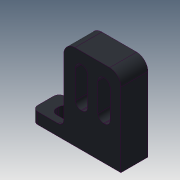
# Autodesk Inventor part: J005556
Saved by Autodesk Inventor 2015 SP1 (Build 190203100, 203)
## iProperties
Created: 2015-12-16
Material: VERO BLACK
Vendor: HHMI: JRC - ID&F
Document SubType Name: Modeling
Designer: ARNOLDJ
Density: 1.17 g/cm^3
Appearance: Black Anodize
Description: NRB ADAPTER ML BRACKET
Project: COMMON
Part Number: J005556
RuleStatus: InUse
AfterDocSave0: file://Part Number Cleaner
LAB/DEPT: COMMON
REQUESTING SCIENTIST: COMMON
SURFACE ROUGHNESS: N/A
DESIGN DEPARTMENT: HHMI: JRC - ID&F
SPECIAL FINISH: NONE
ALTERED ITEM PART NUMBER: N/A
ALTERED ITEM VENDOR: N/A
ALTERED ITEM DESCRIPTION: N/A
Revision Number: -
Autodesk Inventor part; units mm, degrees
sketch "Sketch1" plane through (0, 0, 0) normal (0, 0, 1) x (1, 0, 0)
  line L0 (0, 57.912) -> (0, -9.652) projected
  line L1 (-63.881, 0) -> (36.576, 0) projected
  line L2 (22.225, 48.26) -> (-27.94, 48.26)
  line L3 (-27.94, 48.26) -> (-27.94, 0)
  line L4 (-27.94, 0) -> (22.225, 0)
  line L5 (22.225, 0) -> (22.225, 48.26)
  line L6 (0, 48.26) -> (0, 0) construction
  line L7 (12.7, 48.26) -> (12.7, 0) construction
  line L8 (3.429, 19.305) -> (-3.429, 19.305)
  line L9 (-3.429, 19.305) -> (-3.429, 41.655)
  line L10 (-3.429, 41.655) -> (3.429, 41.655)
  line L11 (3.429, 41.655) -> (3.429, 19.305)
  line L12 (3.429, 19.305) -> (-3.429, 41.655) construction
  line L13 (-3.429, 19.305) -> (3.429, 41.655) construction
  line L14 (16.129, 19.305) -> (9.271, 19.305)
  line L15 (9.271, 19.305) -> (9.271, 41.655)
  line L16 (9.271, 41.655) -> (16.129, 41.655)
  line L17 (16.129, 41.655) -> (16.129, 19.305)
  line L18 (16.129, 19.305) -> (9.271, 41.655) construction
  line L19 (9.271, 19.305) -> (16.129, 41.655) construction
  circle A0 centre (0, 38.48) radius 3.175 construction
  circle A1 centre (0, 30.48) radius 3.175 construction
  line L20 (-27.94, 0) -> (-49.53, 0)
  line L21 (-49.53, 0) -> (-49.53, 7.62)
  line L22 (-49.53, 7.62) -> (-27.94, 7.62)
  line L23 (-27.94, 7.62) -> (-27.94, 0)
  line L24 (-3.9178, 6.35) -> (-23.2802, 6.35)
  line L25 (-23.2802, 6.35) -> (-23.2802, 13.335)
  line L26 (-23.2802, 13.335) -> (-3.9178, 13.335)
  line L27 (-3.9178, 13.335) -> (-3.9178, 6.35)
  line L28 (-3.9178, 6.35) -> (-23.2802, 13.335) construction
  line L29 (-23.2802, 6.35) -> (-3.9178, 13.335) construction
  line L30 (-23.2802, 13.335) -> (-17.0915, 20.955)
  line L31 (-17.0915, 20.955) -> (-10.1065, 20.955)
  line L32 (-10.1065, 20.955) -> (-3.9178, 13.335)
  line L33 (-13.599, 9.8425) -> (-13.599, 20.955) construction
  circle A2 centre (0, 22.48) radius 6.35 construction
  point P0 (0, 0)
  point P1 (0, 25.4)
  point P2 (0, 30.48)
  point P3 (12.7, 30.48)
  point P4 (12.7, 30.48)
  dimension "d0" = 48.26
  dimension "d2" = 6.858
  dimension "d3" = 0
  dimension "d5" = 6.35
  dimension "d6" = 8
  dimension "d27" = 12.7
  dimension "d56" = 41.655
  dimension "d57" = 6.605
  dimension "d58" = 30.48
  dimension "d59" = 7.62
  dimension "d60" = 21.59
  dimension "d61" = 6.985
  dimension "d62" = 6.35
  dimension "d64" = 13.599
  dimension "d81" = 22.225
  dimension "d82" = 27.94
  dimension "d84" = 6.985
  dimension "d85" = 3.4925
  dimension "d86" = 7.62
  dimension "d104" = 12.7
  dimension "d105" = 8
  dimension "d119" = 13.599
  constraints: 64 end point, 10 parallel, 10 point on line, 9 midpoint, 8 perpendicular, 6 horizontal, 3 centre point, 2 coincident, 2 equal length, 1 equal radius, 1 horizontal alignment, 1 tangent
  measures "d0" distance of L2.end L3.end
  measures "d2" distance of L9.end L10.end
  measures "d3" distance between parallel lines of L0 L6
  measures "d5" diameter of A0
  measures "d6" distance of A0.centre A1.centre
  measures "d27" distance of point (0, 30.48) point (12.7, 30.48)
  measures "d56" distance between parallel lines of L4 L10
  measures "d57" distance between parallel lines of L10 L2
  measures "d58" distance from line of L1 A1.centre
  measures "d59" distance of L20.end L21.end
  measures "d60" distance of L21.end L22.end
  measures "d61" distance of L26.end L24.start
  measures "d62" distance between parallel lines of L4 L24
  measures "d64" distance from line of L0 L33.start
  measures "d81" distance between parallel lines of L0 L5
  measures "d82" distance between parallel lines of L3 L0
  measures "d84" distance of L30.end L31.end
  measures "d85" distance from line of L33 L31.end
  measures "d86" distance between parallel lines of L26 L31
  measures "d104" diameter of A2
  measures "d105" distance of A2.centre point (0, 30.48)
  measures "d119" distance from line of L6 L33.start
extrude "Extrusion1" add sketch "Sketch1" along normal blind 15.24 contours L2 L5 L1 L0 L8 L11 L10 | L0 L10 L9 L8 L1 L3 L2 | L24 L25 L26 L27 | L26 L30 L31 L32
ref_plane "Work Plane4" through (-22.225, 7.62, 15.24) normal (0, 1, 0) x (1, 0, 0)
sketch "Sketch4" plane through (-22.225, 7.62, 15.24) normal (0, 1, 0) x (1, 0, 0)
  line L0 (-23.495, 8.255) -> (0, 8.255) projected
  line L1 (-23.495, 8.255) -> (-23.495, -17.78) projected
  line L2 (-23.495, 8.255) -> (-14.605, 8.255)
  line L3 (-14.605, 8.255) -> (-14.605, 0)
  line L4 (-14.605, 0) -> (-23.495, 0)
  line L5 (-23.495, 0) -> (-23.495, 8.255)
  line L6 (44.45, 0) -> (0, 0) projected
  point P0 (22.225, 15.24)
  dimension "d28" = 0
  dimension "d29" = 8.89
  constraints: 8 end point, 2 parallel, 1 horizontal, 1 perpendicular
  measures "d28" distance between parallel lines of L6 L4
  measures "d29" distance between parallel lines of L1 L3
extrude "Extrusion4" [suppressed]
fillet "Fillet1" radius 3.175 8 edges at (-3.429, 19.305, 7.62) (3.429, 19.305, 7.62) (3.429, 41.655, 7.62) (-3.429, 41.655, 7.62) (9.271, 41.655, 7.62) (16.129, 41.655, 7.62) (16.129, 19.305, 7.62) (9.271, 19.305, 7.62)
ref_plane "Work Plane1" through (0, 22.48, 0) normal (-1, 0, 0) x (0, 0, 1)
ref_plane "Work Plane2" through (0, 0, -9.525) normal (0, 0, 1) x (1, 0, 0)
extrude "Extrusion8" cut sketch "Sketch1" along normal up to next contours L24 L25 L26 L27 | L26 L30 L31 L32
ref_plane "Work Plane5" through (-13.599, 6.35, 15.24) normal (1, 0, 0) x (0, 0, -1)
sketch "Sketch7" plane through (22.225, 0, 0) normal (0, -1, 0) x (1, 0, 0)
  line L0 (0, 0) -> (0, 15.24) projected
  line L1 (-50.165, 15.24) -> (0, 15.24) projected
  line L2 (-50.165, 0) -> (0, 0) projected
  line L3 (-71.755, 7.62) -> (0, 7.62) construction
  line L4 (-53.204, 3.81) -> (-68.444, 3.81)
  line L5 (-68.444, 3.81) -> (-68.444, 11.43)
  line L6 (-68.444, 11.43) -> (-53.204, 11.43)
  line L7 (-53.204, 11.43) -> (-53.204, 3.81)
  line L8 (-53.204, 3.81) -> (-68.444, 11.43) construction
  line L9 (-68.444, 3.81) -> (-53.204, 11.43) construction
  line L10 (-43.444, 3.81) -> (-28.204, 3.81)
  line L11 (-28.204, 3.81) -> (-28.204, 11.43)
  line L12 (-28.204, 11.43) -> (-43.444, 11.43)
  line L13 (-43.444, 11.43) -> (-43.444, 3.81)
  line L14 (-43.444, 3.81) -> (-28.204, 11.43) construction
  line L15 (-28.204, 3.81) -> (-43.444, 11.43) construction
  line L16 (-50.165, 0) -> (0, 0) projected
  line L17 (0, 0) -> (0, 15.24) projected
  line L18 (-50.165, 15.24) -> (0, 15.24) projected
  line L19 (-45.5052, 0) -> (-26.1428, 0) projected
  line L20 (-26.1428, 15.24) -> (-45.5052, 15.24) projected
  line L21 (-45.5052, 0) -> (-45.5052, 15.24) projected
  line L22 (-26.1428, 0) -> (-26.1428, 15.24) projected
  line L23 (-35.824, 18.288) -> (-35.824, -3.048) projected
  line L24 (-50.165, 0) -> (-50.165, 15.24) projected
  line L25 (-22.225, 18.288) -> (-22.225, -3.048) projected
  point P0 (-22.225, 0)
  point P1 (-60.824, 7.62)
  point P2 (-35.824, 7.62)
  point P3 (-22.225, 0)
  point P4 (-22.225, 0)
  point P5 (-22.225, 0)
  point P6 (-25.856, 0)
  point P7 (-35.824, 7.62)
  dimension "d69" = 7.62
  dimension "d70" = 15.24
  dimension "d71" = 25
  dimension "d88" = 0
  dimension "d120" = 9.6812
  constraints: 26 end point, 6 midpoint, 4 parallel, 2 equal length, 2 horizontal, 2 perpendicular, 2 point on line, 1 other
  measures "d69" distance of L4.end L5.end
  measures "d70" distance of L5.end L6.end
  measures "d71" distance of point (-60.824, 7.62) point (-35.824, 7.62)
  measures "d88" distance from line of L23 point (-35.824, 7.62)
extrude "Extrusion10" cut sketch "Sketch7" against normal up to surface (6.35 mm away) contours L23 L12 L11 L10 | L10 L13 L12 L23
sketch "Sketch9" plane through (0, 0, 0) normal (0, 0, 1) x (1, 0, 0)
  line L0 (-10.1063, 6.35) -> (-27.94, 6.35)
  line L1 (-27.94, 6.35) -> (-27.94, 48.26)
  line L2 (-27.94, 48.26) -> (-10.1063, 48.26)
  line L3 (-10.1063, 48.26) -> (-10.1063, 6.35)
  line L4 (-3.9178, 6.35) -> (-23.2802, 6.35) projected
  point P0 (0, 0)
  dimension "d101" = 0
  constraints: 8 end point, 2 parallel, 1 horizontal, 1 perpendicular
  measures "d101" distance between parallel lines of L0 L4
extrude "Extrusion12" cut sketch "Sketch9" along normal up to next
fillet "Fillet15" radius 3.175 4 edges at (-5.979, 3.175, 3.81) (-5.979, 3.175, 11.43) (-21.219, 3.175, 11.43) (-21.219, 3.175, 3.81)
sketch "Sketch10" plane through (0, 0, 0) normal (0, 0, -1) x (-1, 0, 0)
  line L0 (10.1065, 20.955) -> (3.9178, 13.335) projected
  line L1 (3.9178, 6.35) -> (3.9178, 13.335) projected
  line L2 (27.94, 6.35) -> (3.9178, 6.35) projected
  line L3 (10.1065, 20.955) -> (10.1065, 6.35)
  line L4 (3.9178, 6.35) -> (27.94, 6.35) projected
  point P0 (0, 0)
  constraints: 2 end point, 1 point on line, 1 vertical
extrude "Extrusion13" add sketch "Sketch10" against normal blind 1.016
sketch "Sketch11" plane through (0, 0, 15.24) normal (0, 0, 1) x (1, 0, 0)
  line L0 (-10.1065, 20.955) -> (-10.1065, 6.35) projected
  line L1 (-10.1063, 20.9547) -> (-3.9178, 13.335) projected
  line L2 (-3.9178, 13.335) -> (-3.9178, 6.35) projected
  line L3 (-3.9178, 6.35) -> (-27.94, 6.35) projected
  line L4 (-10.1063, 20.9547) -> (-10.1065, 6.35)
  point P0 (0, 0)
  constraints: 2 end point
extrude "Extrusion14" add sketch "Sketch11" against normal blind 1.016
fillet "Fillet18" radius 3.175 2 edges at (-3.9178, 9.8425, 1.016) (-3.9178, 9.8425, 14.224)
fillet "Fillet19" radius 3.175 2 edges at (-27.94, 3.175, 0) (-27.94, 3.175, 15.24)
fillet "Fillet20" radius 3.175 2 edges at (-10.1065, 6.35, 14.732) (-10.1065, 6.35, 0.508)
sketch "Sketch12" plane through (0, 0, 0) normal (0, 0, -1) x (-1, 0, 0)
  line L0 (-12.7, 30.48) -> (0, 30.48) construction
  line L1 (0.254, 15.876) -> (-12.954, 15.876)
  line L2 (-19.304, 22.226) -> (-19.304, 38.734)
  line L3 (-12.954, 45.084) -> (0.254, 45.084)
  line L4 (6.604, 38.734) -> (6.604, 22.226)
  line L5 (6.604, 15.876) -> (-19.304, 45.084) construction
  line L6 (-19.304, 15.876) -> (6.604, 45.084) construction
  arc A0 (-12.954, 45.084) -> (-19.304, 38.734) centre (-12.954, 38.734) ccw
  arc A1 (6.604, 38.734) -> (0.254, 45.084) centre (0.254, 38.734) ccw
  arc A2 (0.254, 15.876) -> (6.604, 22.226) centre (0.254, 22.226) ccw
  arc A3 (-19.304, 22.226) -> (-12.954, 15.876) centre (-12.954, 22.226) ccw
  point P0 (0, 0)
  point P1 (-6.35, 30.48)
  dimension "d113" = 6.604
  dimension "d114" = 14.604
  dimension "d115" = 6.35
  constraints: 14 end point, 8 point on circle, 8 point on line, 8 tangent, 4 centre point, 3 equal radius, 3 midpoint, 2 horizontal, 2 parallel, 1 perpendicular
  measures "d113" distance from line of L2 L0.start
  measures "d114" distance from line of L1 L0.start
  measures "d115" radius of A0
extrude "Extrusion15" cut sketch "Sketch12" against normal blind 5.08
fillet "Fillet21" radius 6.35 2 edges at (22.225, 48.26, 7.62) (-10.1063, 48.26, 7.62)
equation "\"d85\" = 0.5 * d84"
body "Solid1"
